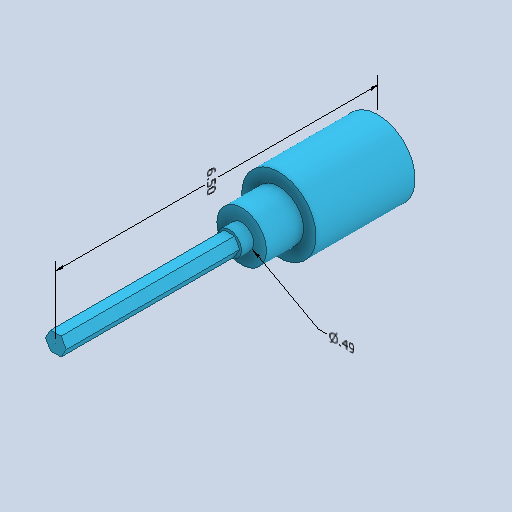
# Autodesk Inventor part: 3_8x6_5-inchHexShaft
Saved by Autodesk Inventor 2022.1 (Build 261234000, 234)
## iProperties
Created: 2020-11-17
Part Number: 3_8x6_5-inchHexShaft
Material: PC/ABS Plastic
Document SubType Name: Modeling
Designer: robst
Density: 0.357273 g/cm^3
Appearance: Turquoise
Author: robst
Autodesk Inventor part; units mm, degrees
ref_plane "YZ Plane" through (0, 0, 0) normal (1, 0, 0) x (0, 1, 0)
ref_plane "XZ Plane" through (0, 0, 0) normal (0, 1, 0) x (-1, 0, 0)
ref_plane "XY Plane" through (0, 0, 0) normal (0, 0, 1) x (1, 0, 0)
sketch "Sketch1" plane through (0, 0, 0) normal (0, 0, 1) x (1, 0, 0)
  line L0 (5.4993, 0) -> (2.7496, -4.7625)
  line L1 (2.7496, -4.7625) -> (-2.7496, -4.7625)
  line L2 (-2.7496, -4.7625) -> (-5.4993, 0)
  line L3 (-5.4993, 0) -> (-2.7496, 4.7625)
  line L4 (-2.7496, 4.7625) -> (2.7496, 4.7625)
  line L5 (2.7496, 4.7625) -> (5.4993, 0)
  circle A0 centre (0, 0) radius 0.0127
  dimension "d0" = 9.525
  dimension "d6" = 0.0254
  constraints: 12 end point, 2 coincident, 1 centre point, 1 horizontal, 13 other
  measures "d0" distance between parallel lines of L1 L4
  measures "d6" diameter of A0
extrude "Extrusion2" add sketch "Sketch1" along normal mid plane 114.3
sketch "Sketch4" plane through (0, 0, -57.15) normal (0, 0, -1) x (-1, 0, 0)
  circle A0 centre (0, 0) radius 0.0127 projected
  circle A1 centre (0, 0) radius 12.7
  dimension "d10" = 25.4
  constraints: 1 centre point, 1 coincident
  measures "d10" diameter of A1
extrude "Extrusion4" add sketch "Sketch4" against normal blind 19.05
thicken "Reduce Hex Shaft" operation add thickness 0.127 both sides no extend neighbours yes toward (0, -1, 0) faces at (0.9165, 4.7625, -6.35) (4.5827, 1.5875, -6.35) (3.6662, -3.175, -6.35) (-3.6662, 3.175, -6.35) (-4.5827, -1.5875, -6.35) (-0.9165, -4.7625, -6.35)
sketch "Sketch5" plane through (0, 0, -38.1) normal (0, 0, 1) x (1, 0, 0)
  circle A0 centre (0, 0) radius 6.35
  dimension "d15" = 12.7
  constraints: 1 centre point, 1 coincident
  measures "d15" diameter of A0
extrude "Extrusion5" add sketch "Sketch5" along normal blind 6.35
thicken "Reduce Base Bushing" operation add thickness 0.127 both sides no extend neighbours yes toward (-0.9967573, 0.0804666, 0) faces at (6.3294, -0.511, -33.8667)
sketch "Sketch8" plane through (0, 0, -57.15) normal (0, 0, -1) x (-1, 0, 0)
  circle A0 centre (0, 0) radius 19.05
  dimension "d28" = 38.1
  constraints: 1 centre point, 1 coincident
  measures "d28" diameter of A0
extrude "Extrusion7" add sketch "Sketch8" along normal blind 50.8
equation "\"d0\" = hexSize"
equation "\"d4\" = length"
equation "\"d13\" = printOffset"
equation "\"d14\" = printOffset"
equation "\"d15\" = bushingForBaseHole"
equation "\"d16\" = sideOfBase"
equation "\"d20\" = printOffset"
equation "\"d21\" = printOffset"
equation "\"hexSize\" = 9.525"
equation "\"length\" = 114.3"
equation "\"printOffset\" = 0.127"
equation "\"bushingForBaseHole\" = 12.7"
equation "\"sideOfBase\" = 6.35"
body "Solid2"
